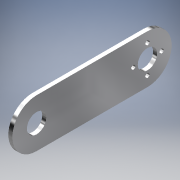
# Autodesk Inventor part: Module Plate
Saved by Autodesk Inventor 2019.4 (Build 234330000, 330)
## iProperties
Created: 2019-12-31
Part Number: Module Plate
Material: Aluminum 6061
Document SubType Name: Modeling
Designer: Mark
Mass: 137.25 g
Surface Area: 234.038 cm^2
Volume: 50.8333 cm^3
Density: 2.7 g/cm^3
Appearance: Aluminum - Flat
Author: Mark
Autodesk Inventor part; units mm, degrees
ref_plane "YZ Plane" through (0, 0, 0) normal (1, 0, 0) x (0, 1, 0)
ref_plane "XZ Plane" through (0, 0, 0) normal (0, 1, 0) x (-1, 0, 0)
ref_plane "XY Plane" through (0, 0, 0) normal (0, 0, 1) x (1, 0, 0)
sketch "Sketch1" plane through (0, 0, 0) normal (1, 0, 0) x (0, 1, 0)
  circle A0 centre (0, 0) radius 12
  circle A1 centre (0, -137.4) radius 12
  line L0 (0, 0) -> (0, -137.4)
  line L1 (0, 0) -> (137.4, 0) construction
  line L2 (0, 0) -> (0, -137.4) construction
  line L3 (-30, 0) -> (-30, -137.4)
  line L4 (30, -137.4) -> (30, 0)
  arc A2 (30, 0) -> (-30, 0) centre (0, 0) ccw
  arc A3 (-30, -137.4) -> (30, -137.4) centre (0, -137.4) ccw
  circle A4 centre (0, -137.4) radius 17.5 construction
  line L5 (0, -137.4) -> (17.5, -137.4) construction
  line L6 (0, -137.4) -> (17.5, -137.4) construction
  circle A5 centre (17.5, -137.4) radius 2.65
  line L7 (0, -137.4) -> (0, -119.9) construction
  circle A6 centre (0, -119.9) radius 2.65
  line L8 (0, -137.4) -> (-17.5, -137.4) construction
  circle A7 centre (-17.5, -137.4) radius 2.65
  line L9 (0, -137.4) -> (0, -154.9) construction
  circle A8 centre (0, -154.9) radius 2.65
  point P0 (0, -68.7)
  dimension "d9" = 35
  dimension "d0" = 24
  dimension "d1" = 24
  dimension "d4" = 90
  dimension "d5" = 137.4
  dimension "d6" = 60
  dimension "d10" = 0
  dimension "d11" = 5.3
  dimension "d14" = 360
  constraints: 22 end point, 8 centre point, 4 point on circle, 4 tangent, 3 coincident, 2 equal length, 2 horizontal, 2 vertical, 1 horizontal alignment, 1 midpoint, 1 parallel, 23 other
  measures "d0" diameter of A0
  measures "d1" diameter of A1
  measures "d4" angle of L0 L1
  measures "d5" distance of L0.start L0.end
  measures "d6" diameter of A3
  measures "d10" distance between parallel lines of L5 L6
  measures "d11" diameter of A5
extrude "Extrusion1" add sketch "Sketch1" along normal blind 5
body "Solid1"
